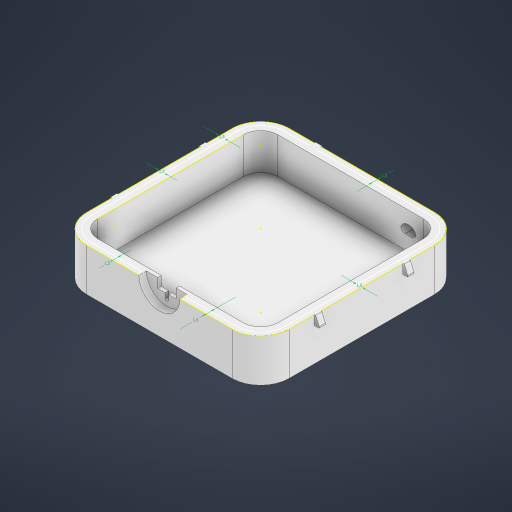
# Autodesk Inventor part: enclosure_down
Saved by Autodesk Inventor 2024.1 (Build 281209000, 209)
## iProperties
Created: 2023-07-19
Part Number: enclosure_down
Material: ABS Plastic
Document SubType Name: Modeling
Designer: LabTel_Admin
Density: 1.06 g/cm^3
Appearance: Smooth - White
Author: LabTel_Admin
Autodesk Inventor part; units mm, degrees
ref_plane "YZ Plane" through (0, 0, 0) normal (1, 0, 0) x (0, 1, 0)
ref_plane "XZ Plane" through (0, 0, 0) normal (0, 1, 0) x (-1, 0, 0)
ref_plane "XY Plane" through (0, 0, 0) normal (0, 0, 1) x (1, 0, 0)
sketch "Sketch1" plane through (0, 0, 0) normal (0, 1, 0) x (-1, 0, 0)
  line L0 (-23, -32) -> (23, -32)
  line L1 (32, -23) -> (32, 23)
  line L2 (23, 32) -> (-23, 32)
  line L3 (-32, 23) -> (-32, -23)
  line L4 (-32, -32) -> (32, 32) construction
  line L5 (32, -32) -> (-32, 32) construction
  arc A0 (32, 23) -> (23, 32) centre (23, 23) ccw
  arc A1 (23, -32) -> (32, -23) centre (23, -23) ccw
  arc A2 (-32, -23) -> (-23, -32) centre (-23, -23) ccw
  arc A3 (-23, 32) -> (-32, 23) centre (-23, 23) ccw
  line L6 (28.5, 23) -> (28.5, -23)
  arc A4 (23, -28.5) -> (28.5, -23) centre (23, -23) ccw
  line L7 (23, -28.5) -> (-23, -28.5)
  arc A5 (-28.5, -23) -> (-23, -28.5) centre (-23, -23) ccw
  line L8 (-28.5, -23) -> (-28.5, 23)
  arc A6 (-23, 28.5) -> (-28.5, 23) centre (-23, 23) ccw
  line L9 (-23, 28.5) -> (23, 28.5)
  arc A7 (28.5, 23) -> (23, 28.5) centre (23, 23) ccw
  point P0 (0, 0)
  point P1 (32, 0)
  point P2 (31.5, 26.5247)
  dimension "d0" = 64
  dimension "d1" = 64
  dimension "d3" = 9
  dimension "d4" = 9
  dimension "d5" = 3.5
  constraints: 20 end point, 16 point on circle, 8 centre point, 8 point on line, 8 tangent, 4 parallel, 3 midpoint, 2 equal radius, 2 perpendicular, 1 horizontal, 7 other
  measures "d0" distance of L5.end L4.end
  measures "d1" distance of L4.end L5.start
  measures "d3" radius of A0
  measures "d4" radius of A1
  measures "d5" distance between parallel lines of L1 L6
extrude "Extrusion1" add sketch "Sketch1" along normal blind 2 contours L6 A4 L7 A5 L8 A6 L9 A7
extrude "Extrusion2" add sketch "Sketch1" along normal blind 13.5
sketch "Sketch2" plane through (-23, 0, 32) normal (0, 0, 1) x (1, 0, 0)
  line L0 (0, 13.5) -> (46, 13.5) projected
  arc A0 (16.5, 13.5) -> (29.5, 13.5) centre (23, 13.5) ccw
  line L1 (16.5, 13.5) -> (29.5, 13.5)
  point P0 (23, 0)
  dimension "d10" = 13
  constraints: 2 end point, 2 point on circle, 2 point on line, 1 centre point, 1 collinear, 1 midpoint
  measures "d10" diameter of A0
extrude "Extrusion3" cut sketch "Sketch2" against normal blind 2.4
sketch "Sketch3" plane through (-23, 0, 29.6) normal (0, 0, 1) x (1, 0, 0)
  line L0 (25.9, 10.5) -> (20.1, 10.5)
  line L1 (20.1, 10.5) -> (20.1, 13.5)
  line L2 (25.9, 13.5) -> (25.9, 10.5)
  line L3 (16.5, 13.5) -> (29.5, 13.5) projected
  line L4 (25.9, 10.5) -> (23, 13.5) construction
  line L5 (20.1, 10.5) -> (25.9, 16.5) construction
  line L6 (20.1, 13.5) -> (25.9, 13.5)
  line L7 (23.5, 10.5) -> (23.5, 9)
  line L8 (23, 8.5) -> (23, 8.5)
  line L9 (22.5, 9) -> (22.5, 10.5)
  line L10 (23, 10.5) -> (23.5, 8.5) construction
  line L11 (23, 10.5) -> (22.5, 8.5) construction
  arc A0 (23, 8.5) -> (23.5, 9) centre (23, 9) ccw
  arc A1 (22.5, 9) -> (23, 8.5) centre (23, 9) ccw
  point P0 (23, 0)
  dimension "d13" = 6
  dimension "d15" = 1
  dimension "d17" = 0.5
  constraints: 22 end point, 8 point on line, 5 midpoint, 4 point on circle, 4 tangent, 2 centre point, 2 parallel, 1 concentric, 1 horizontal, 1 perpendicular
  measures "d13" distance of L5.end L0.start
  measures "d15" distance of L10.end L11.end
  measures "d17" radius of A0
extrude "Extrusion4" cut sketch "Sketch3" against normal blind 2
sketch "Sketch4" plane through (32, 0, 23) normal (1, 0, 0) x (0, 0, -1)
  line L0 (46, 13.5) -> (0, 13.5) projected
  line L1 (8, 13.5) -> (10, 13.5)
  line L2 (10, 13.5) -> (10, 10.5)
  line L3 (10, 10.5) -> (8, 10.5)
  line L4 (8, 10.5) -> (8, 13.5)
  line L5 (0, 0) -> (0, 13.5) projected
  line L6 (23, 0) -> (23, 18.3327) construction
  line L7 (38, 13.5) -> (36, 13.5)
  line L8 (36, 13.5) -> (36, 10.5)
  line L9 (36, 10.5) -> (38, 10.5)
  line L10 (38, 10.5) -> (38, 13.5)
  point P0 (10, 13.5)
  dimension "d20" = 2
  dimension "d21" = 3
  dimension "d22" = 8
  constraints: 18 end point, 4 symmetric about line, 2 parallel, 2 perpendicular, 1 horizontal, 1 point on line
  measures "d20" distance of L2.end L3.end
  measures "d21" distance of L1.end L2.end
  measures "d22" distance between parallel lines of L5 L4
extrude "Extrusion5" add sketch "Sketch4" along normal blind 1.5
sketch "Sketch5" plane through (32, 10.5, 15) normal (0, 0, 1) x (1, 0, 0)
  line L0 (1.5, 0) -> (1.5, 3) projected
  line L1 (0, 3) -> (-9, 3) projected
  line L2 (1.5, 0.4) -> (0.4, 3)
  line L3 (0, 3) -> (1.5, 3) projected
  line L4 (0, -10.5) -> (0, 3) projected
  line L5 (0.4, 3) -> (1.5, 3)
  line L6 (1.5, 0.4) -> (1.5, 3)
  point P0 (-32, -10.5)
  dimension "d25" = 0.4
  dimension "d26" = 0.4
  constraints: 6 end point, 2 point on line, 1 collinear, 1 perpendicular
  measures "d25" distance of L0.start L2.start
  measures "d26" distance from line of L4 L2.end
extrude "Extrusion6" cut sketch "Sketch5" against normal blind 50
mirror "Mirror1" about plane through (0, 0, 0) normal (1, 0, 0) of "Extrusion6", "Extrusion5"
sketch "Sketch7" plane through (23, 0, -32) normal (0, 0, -1) x (-1, 0, 0)
  line L0 (46, 13.5) -> (0, 13.5) projected
  line L1 (38, 13.5) -> (36, 13.5)
  line L2 (36, 13.5) -> (36, 10.5)
  line L3 (36, 10.5) -> (38, 10.5)
  line L4 (38, 10.5) -> (38, 13.5)
  line L5 (46, 0) -> (46, 13.5) projected
  point P0 (23, 0)
  point P1 (30, 13.5)
  dimension "d34" = 2
  dimension "d35" = 3
  dimension "d36" = 8
  constraints: 8 end point, 2 parallel, 1 horizontal, 1 perpendicular, 1 point on line
  measures "d34" distance of L3.end L2.end
  measures "d35" distance of L2.end L1.end
  measures "d36" distance between parallel lines of L5 L4
extrude "Extrusion8" add sketch "Sketch7" along normal blind 1.5
sketch "Sketch8" plane through (-15, 10.5, -32) normal (-1, 0, 0) x (0, 0, 1)
  line L0 (-1.5, 3) -> (-1.5, 0) projected
  line L1 (-1.5, 0.4) -> (-0.4, 3)
  line L2 (0, 3) -> (-1.5, 3) projected
  line L3 (0, 0) -> (-1.5, 0) projected
  line L4 (0, -10.5) -> (0, 3) projected
  line L5 (-0.4, 3) -> (-1.5, 3)
  line L6 (-1.5, 3) -> (-1.5, 0.4)
  line L7 (-0.4, 3) -> (-0.4, 1.4673) construction
  point P0 (32, -10.5)
  dimension "d39" = 0.4
  dimension "d40" = 0.4
  constraints: 8 end point, 2 point on line, 1 collinear, 1 horizontal, 1 vertical
  measures "d39" distance from line of L3 L1.start
  measures "d40" distance from line of L4 L1.end
extrude "Extrusion9" cut sketch "Sketch8" against normal blind 3 contours L2 L1 L0
sketch "Sketch9" plane through (23, 0, -32) normal (0, 0, -1) x (-1, 0, 0)
  line L0 (5.7297, 6.5453) -> (3.7297, 6.5453)
  line L1 (4.7297, 9.5453) -> (4.7297, 9.5453)
  arc A0 (7.1651, 7.6099) -> (4.7297, 9.5453) centre (4.7297, 7.0453) ccw
  arc A1 (5.7297, 6.5453) -> (7.1651, 7.6099) centre (5.7297, 8.0453) ccw
  arc A2 (2.2943, 7.6099) -> (3.7297, 6.5453) centre (3.7297, 8.0453) ccw
  arc A3 (4.7297, 9.5453) -> (2.2943, 7.6099) centre (4.7297, 7.0453) ccw
  point P0 (23, 0)
  point P1 (2.2297, 6.5453)
  point P2 (7.2297, 6.5453)
  point P3 (2.2297, 9.5453)
  point P4 (4.7297, 9.5453)
  dimension "d45" = 3
  dimension "d46" = 5
  dimension "d47" = 2.5
  dimension "d48" = 1.5
  dimension "d49" = 1.5
  dimension "d50" = 2.5
  constraints: 8 point on circle, 4 centre point, 4 end point, 4 tangent, 3 point on line, 1 parallel
  measures "d45" distance of point (2.23, 6.545) point (2.23, 9.545)
  measures "d46" distance of point (7.23, 6.545) point (2.23, 6.545)
  measures "d47" radius of A0
  measures "d48" radius of A1
  measures "d49" radius of A2
  measures "d50" radius of A3
extrude "Extrusion10" cut sketch "Sketch9" against normal blind 3.5
sketch "Sketch11" plane through (0, 13.5, 0) normal (0, 1, 0) x (1, 0, 0)
  line L0 (-32, 13) -> (-32, -13) projected
  line L1 (-32, -15) -> (-32, -23) projected
  arc A0 (-32, -23) -> (-23, -32) centre (-23, -23) ccw projected
  line L2 (-23, -32) -> (-6.5, -32) projected
  line L3 (6.5, -32) -> (23, -32) projected
  arc A1 (23, -32) -> (32, -23) centre (23, -23) ccw projected
  line L4 (32, -23) -> (32, -15) projected
  line L5 (32, -13) -> (32, 13) projected
  line L6 (32, 15) -> (32, 23) projected
  arc A2 (32, 23) -> (23, 32) centre (23, 23) ccw projected
  line L7 (23, 32) -> (-13, 32) projected
  line L8 (-15, 32) -> (-23, 32) projected
  arc A3 (-23, 32) -> (-32, 23) centre (-23, 23) ccw projected
  line L9 (-32, 23) -> (-32, 15) projected
  line L10 (6.5, -30.5) -> (23, -30.5)
  arc A4 (23, -30.5) -> (30.5, -23) centre (23, -23) ccw
  line L11 (30.5, -23) -> (30.5, -15)
  line L12 (-6.5, -30.5) -> (-23, -30.5)
  arc A5 (-30.5, -23) -> (-23, -30.5) centre (-23, -23) ccw
  line L13 (-30.5, -23) -> (-30.5, -15)
  line L14 (-30.5, 13) -> (-30.5, -13)
  line L15 (-30.5, 15) -> (-30.5, 23)
  arc A6 (-23, 30.5) -> (-30.5, 23) centre (-23, 23) ccw
  line L16 (-23, 30.5) -> (-15, 30.5)
  line L17 (-13, 30.5) -> (23, 30.5)
  arc A7 (30.5, 23) -> (23, 30.5) centre (23, 23) ccw
  line L18 (30.5, 23) -> (30.5, 15)
  line L19 (30.5, -13) -> (30.5, 13)
  line L20 (30.5, -15) -> (30.5, -13)
  line L21 (30.5, 13) -> (30.5, 15)
  line L22 (-28.5, 23) -> (-28.5, -23) projected
  line L23 (-30.5, 15) -> (-30.5, 13)
  line L24 (-30.5, -15) -> (-30.5, -13)
  line L25 (6.5, -29.6) -> (6.5, -32) projected
  line L26 (6.5, -30.5) -> (6.5, -29.6)
  point P0 (0, 0)
  dimension "d53" = 1.5
  dimension "d54" = 1.5
  dimension "d55" = 1.5
  dimension "d56" = 1.5
  dimension "d57" = 1.5
  dimension "d58" = 1.5
  constraints: 30 end point, 8 point on circle, 4 centre point, 3 collinear, 2 parallel, 8 other
  measures "d53" distance between parallel lines of L3 L10
  measures "d54" distance between parallel lines of L2 L12
  measures "d55" distance between parallel lines of L0 L14
  measures "d56" distance between parallel lines of L9 L15
  measures "d57" distance between parallel lines of L7 L17
  measures "d58" distance between parallel lines of L5 L19
body "Solid1"
